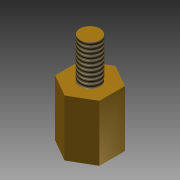
# Autodesk Inventor part: Motherboard Standoff 11mm M3x0.5
Saved by Autodesk Inventor 2016 (Build 200138000, 138)
## iProperties
Created: 2011-08-02
Part Number: Motherboard Standoff 11mm M3x0.5
Material: Generic
Document SubType Name: Modeling
Designer: darkz
Density: 1 g/cm^3
Mass: 0.18829 g
Surface Area: 2.56448 cm^2
Volume: 0.18829 cm^3
Appearance: Default
Author: darkz
Autodesk Inventor part; units mm, degrees
ref_plane "YZ Plane" through (0, 0, 0) normal (1, 0, 0) x (0, 1, 0)
ref_plane "XZ Plane" through (0, 0, 0) normal (0, 1, 0) x (-1, 0, 0)
ref_plane "XY Plane" through (0, 0, 0) normal (0, 0, 1) x (1, 0, 0)
sketch "Sketch1" plane through (0, 0, 0) normal (0, 0, 1) x (1, 0, 0)
  line L0 (0, 4.4456) -> (0, -4.4456) projected
  line L1 (-3.85, 0) -> (3.85, 0) projected
  circle A0 centre (0, 0) radius 1.25
  line L2 (0, 3.1754) -> (2.75, 1.5877)
  line L3 (2.75, 1.5877) -> (2.75, -1.5877)
  line L4 (2.75, -1.5877) -> (0, -3.1754)
  line L5 (0, -3.1754) -> (-2.75, -1.5877)
  line L6 (-2.75, -1.5877) -> (-2.75, 1.5877)
  line L7 (-2.75, 1.5877) -> (0, 3.1754)
  dimension "d0" = 2.5
  dimension "d1" = 5.5
  constraints: 12 end point, 2 coincident, 1 centre point, 1 point on line, 13 other
  measures "d0" diameter of A0
  measures "d1" distance between parallel lines of L7 L4
extrude "Extrusion1" add sketch "Sketch1" along normal mid plane 12
sketch "Sketch2" plane through (0, 0, -6) normal (0, 0, -1) x (-1, 0, 0)
  circle A0 centre (0, 0) radius 1.25
  dimension "d4" = 2.5
  constraints: 1 centre point, 1 coincident
  measures "d4" diameter of A0
extrude "Extrusion2" cut sketch "Sketch2" against normal blind 4
sketch "Sketch3" plane through (2.75, -1.5877, 6) normal (1, 0, 0) x (0, 0, -1)
  line L0 (0, 3.1754) -> (0, 0) projected
  line L1 (12, 0) -> (0, 0) projected
  line L2 (12, 0) -> (12, 3.1754) projected
  line L3 (12, 3.1754) -> (0, 3.1754) projected
  line L4 (6, 0) -> (6, 3.1754)
  point P0 (6, 1.5877)
  constraints: 2 end point, 2 midpoint
sketch "Sketch4" plane through (0, 0, 6) normal (0, 0, 1) x (1, 0, 0)
  line L0 (0, 3.1754) -> (2.75, 1.5877) projected
  line L1 (-2.75, 1.5877) -> (0, 3.1754) projected
  line L2 (-2.75, -1.5877) -> (-2.75, 1.5877) projected
  line L3 (0, -3.1754) -> (-2.75, -1.5877) projected
  line L4 (2.75, -1.5877) -> (0, -3.1754) projected
  line L5 (2.75, 1.5877) -> (2.75, -1.5877) projected
  circle A0 centre (0, 0) radius 1.25
  dimension "d7" = 2.5
  constraints: 1 centre point, 1 coincident
  measures "d7" diameter of A0
extrude "Extrusion3" cut sketch "Sketch4" against normal blind 5
thread "Thread1" size "M3x0.5" class "6H" standard "ANSI Metric M Profile" full length
thread "Thread2" size "M3x0.5" class "6g" standard "ANSI Metric M Profile" full length
body "Solid1"
